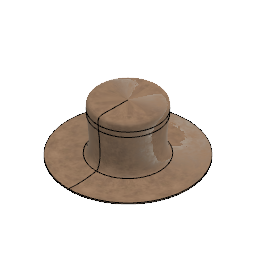
32-leather hat v1 (Autodesk Fusion 360 design; units mm, degrees)
Autodesk Fusion 360 part; units mm, degrees
sketch "Sketch1" plane through (0, 0, 0) normal (0, 0, 1) x (1, 0, 0)
  line L0 (100, 14.705) -> (100, 16.7231)
  line L1 (52.1792, 14.2271) -> (52.4763, 14.3829)
  spline S0 degree 5 poles (52.4763, 14.3829) (53.5566, 14.5598) (56.961, 15.1131) (62.6816, 16.0073) (70.697, 17.0821) (80.2228, 17.8215) (88.6122, 17.7915) (94.6821, 17.3616) (98.4706, 16.9264) (100, 16.7231) knots 0.676771 0.676771 0.676771 0.676771 0.676771 0.676771 0.7 0.75 0.8 0.85 0.883946 0.883946 0.883946 0.883946 0.883946 0.883946
  line L2 (47.6277, 13.5887) -> (57.3249, 15.177)
  line L3 (95.2002, 17.3612) -> (104.7998, 16.0851)
  spline S1 degree 3 poles (53.1076, 12.4557) (59.1362, 13.4383) (65.1185, 14.36) (71.0393, 14.9528) (80.1376, 15.8636) (89.0962, 15.9871) (97.9394, 14.9639) (98.6269, 14.8844) (99.3138, 14.7981) (100, 14.705) knots 0.678102 0.678102 0.678102 0.678102 0.756049 0.756049 0.756049 0.875825 0.875825 0.875825 0.885138 0.885138 0.885138 0.885138
  line L4 (0, 0) -> (0, -100)
  spline S2 degree 3 poles (52.1792, 14.2271) (50.4545, 13.3233) (49.0984, 11.7935) (48.0812, 9.8625) (46.4573, 6.7798) (45.5787, 2.5891) (45.1691, -2.6218) (44.7752, -7.6321) (44.8484, -13.6003) (45.2048, -19.8879) (45.6525, -27.7884) (46.5551, -36.1262) (47.2908, -43.0931) (47.7725, -47.6545) (48.1741, -51.6256) (48.2775, -54.6436) (48.3591, -57.0234) (48.2315, -58.8071) (47.9224, -59.8999) (47.7016, -60.6809) (47.4395, -61.0931) (47.0857, -61.4221) (46.7201, -61.7623) (46.1708, -62.0616) (45.2352, -62.3049) (43.3781, -62.7878) (40.1595, -62.921) (35.7356, -62.8899) (29.4451, -62.8456) (20.6695, -62.5696) (9.4402, -62.5532) (6.4647, -62.5489) (3.3175, -62.562) (0, -62.5938) knots 0 0 0 0 0.06187 0.06187 0.06187 0.160645 0.160645 0.160645 0.255617 0.255617 0.255617 0.374953 0.374953 0.374953 0.453083 0.453083 0.453083 0.514692 0.514692 0.514692 0.558717 0.558717 0.558717 0.604228 0.604228 0.604228 0.694568 0.694568 0.694568 0.823028 0.823028 0.823028 0.857066 0.857066 0.857066 0.857066
  spline S3 degree 5 poles (53.1076, 12.4557) (52.4825, 12.1281) (51.3119, 11.2772) (49.7953, 9.4139) (48.2535, 5.7506) (47.1201, -0.7466) (46.7415, -8.978) (47.0206, -18.5211) (47.7864, -28.672) (48.8076, -38.6092) (49.8013, -47.5148) (50.4411, -54.7212) (50.3666, -59.8284) (49.1868, -62.8917) (46.5075, -64.3985) (41.9979, -64.9325) (35.4449, -64.9355) (26.7256, -64.7306) (17.6604, -64.5741) (9.6815, -64.5345) (3.7325, -64.5579) (0.416, -64.5862) (0, -64.5899) knots 0 0 0 0 0 0 0.05 0.1 0.15 0.2 0.25 0.3 0.35 0.4 0.45 0.5 0.55 0.6 0.65 0.7 0.75 0.8 0.85 0.857126 0.857126 0.857126 0.857126 0.857126 0.857126
  line L5 (21.0857, -64.3989) -> (-21.0857, -64.7809)
  line L6 (48.1945, -52.9326) -> (50.1982, -52.9326)
  line L7 (46.1786, -32.248) -> (48.1833, -32.248)
  line L8 (47.4663, -44.7664) -> (49.477, -44.7664)
  point P0 (69.5784, 16.812)
  point P1 (46.9404, -7.1576)
  point P2 (50.2743, -57.4271)
  point P3 (46.2746, -64.0853)
  constraint vertical L0
  constraint midpoint L1.end L2
  constraint midpoint L0.end L3
  constraint coincident L4.start origin
  constraint vertical L4
  constraint coincident L4 S2.end
  constraint coincident L4 S3.end
  constraint midpoint S3.end L5
  constraint coincident S2 L6.start
  constraint coincident S3 L6.end
  constraint horizontal L6
  constraint coincident S2 L7.start
  constraint coincident S3 L7.end
  constraint parallel L6 L7
  constraint coincident S2 L8.start
  constraint coincident S3 L8.end
  constraint parallel L6 L8
revolve "Revolve1" add sketch "Sketch1" angle 360 about axis through (0, 0, 0) along (0, -1, 0) makes body 1
revolve "Revolve2" cut sketch "Sketch1" angle 360 about axis through (0, 0, 0) along (0, -1, 0) contours S2 S3 L6 L8 bodies 1 makes body 2 at (-27.0556, -64.7941, 11.4049)
revolve "Revolve3" add sketch "Sketch1" angle 360 about axis through (0, 0, 0) along (0, -1, 0) separate body contours S2 S3 L6 L8 makes body 3
move_body "Move2" bodies 3 2 1 to x (0, 0, 1) y (0, -1, 0) z (1, 0, 0) at (-63.5808, -28.148, 63.5808)
combine "Combine1" operation add target body 1 tool bodies 3 2
move_body "Move1" [suppressed]
